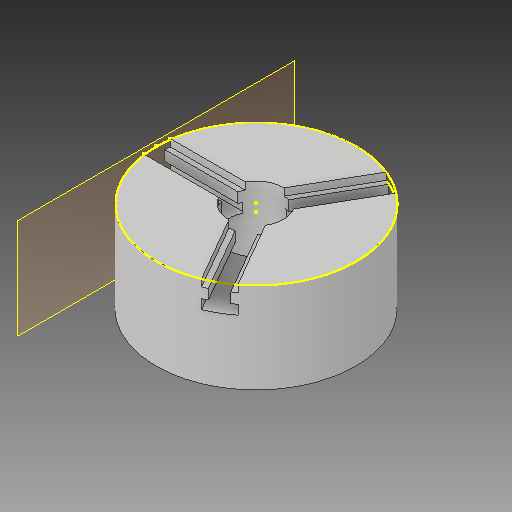
# Autodesk Inventor part: 3 jaww
Saved by Autodesk Inventor 2018 (Build 220112000, 112)
## iProperties
Created: 2017-06-20
Part Number: 3 jaww
Material: Generic
Document SubType Name: Modeling
Designer: M228854
Density: 1 g/cm^3
Appearance: Default
Author: M228854
Autodesk Inventor part; units mm, degrees
ref_plane "XZ Plane" through (0, 0, 0) normal (0, 1, 0) x (-1, 0, 0)
ref_plane "XY Plane" through (0, 0, 0) normal (0, 0, 1) x (1, 0, 0)
sketch "Sketch1" plane through (0, 0, 0) normal (0, 1, 0) x (-1, 0, 0)
  circle A0 centre (0, 0) radius 99.7
  constraints: 1 centre point, 1 coincident
extrude "Extrusion1" add sketch "Sketch1" along normal blind 90.9
sketch "Sketch2" plane through (0, 90.9, 0) normal (0, 1, 0) x (1, 0, 0)
  circle A0 centre (0, 0) radius 27.56
  dimension "d3" = 55.12
  constraints: 1 centre point, 1 coincident
  measures "d3" diameter of A0
extrude "Extrusion2" cut sketch "Sketch2" against normal blind 90.9
sketch "Sketch3" plane through (0, 90.9, 0) normal (0, 1, 0) x (1, 0, 0)
  circle A0 centre (0, 0) radius 99.7 projected
  line L0 (-99.7, 0) -> (-98.8062, 13.32)
  line L1 (-98.8062, 13.32) -> (-24.1274, 13.32)
  circle A1 centre (0, 0) radius 27.56 projected
  line L2 (-99.7, 0) -> (-98.8062, -13.32)
  line L3 (-98.8062, -13.32) -> (-24.1274, -13.32)
  line L4 (37.8676, -92.2287) -> (0.5282, -27.5549)
  line L5 (49.85, -86.3427) -> (37.8676, -92.2287)
  line L6 (49.85, -86.3427) -> (60.9386, -78.9087)
  line L7 (60.9386, -78.9087) -> (23.5992, -14.2349)
  line L8 (60.9386, 78.9087) -> (23.5992, 14.2349)
  line L9 (49.85, 86.3427) -> (60.9386, 78.9087)
  line L10 (49.85, 86.3427) -> (37.8676, 92.2287)
  line L11 (37.8676, 92.2287) -> (0.5282, 27.5549)
  line L12 (-24.1274, 13.32) -> (-24.1274, -13.32)
  line L13 (0.5282, 27.5549) -> (23.5992, 14.2349)
  line L14 (23.5992, -14.2349) -> (0.5282, -27.5549)
  dimension "d6" = 13.35
  dimension "d15" = 360
  constraints: 30 end point, 5 point on circle, 2 horizontal, 1 perpendicular, 1 vertical, 28 other
  measures "d6" distance of L0.start L0.end
extrude "Extrusion6" cut sketch "Sketch3" against normal blind 7.18 contours L8 A1 L11 L10 L9 | L6 L5 L4 A1 L7 | L13 A1 | A1 L14 | L1 A1 L3 L2 L0
sketch "Sketch7" plane through (49.85, 83.72, -86.3427) normal (-0.5568593, 0, 0.8306069) x (0.8306069, 0, 0.5568593)
  line L0 (13.35, 7.18) -> (0, 7.18) projected
  line L1 (13.35, 0) -> (13.35, 7.18) projected
  line L2 (0, 7.18) -> (13.35, 7.18)
  line L3 (13.35, 0) -> (18.3498, 0) projected
  line L4 (13.35, 7.18) -> (13.35, 0)
  line L5 (0, 7.18) -> (0, 0) projected
  line L6 (13.35, 0) -> (0, 0)
  line L7 (0, 0) -> (0, 6.2119)
  line L8 (0, 7.18) -> (-13.2303, 7.18) projected
  line L9 (-13.2303, 4.6736) -> (0, 7.18)
  line L10 (0, 7.18) -> (0, 0)
  line L11 (-13.2303, -2.9965) -> (-13.2303, 4.6736)
  line L12 (-13.2303, 0) -> (-13.2303, 7.18) projected
  point P0 (6.675, -83.72)
  constraints: 14 end point, 3 perpendicular, 2 collinear, 1 point on line
extrude "Extrusion7" cut sketch "Sketch7" against normal blind 10 contours L1 L6 L5 L0
sketch "Sketch8" plane through (37.8676, 83.72, -92.2287) normal (-0.440897, 0, 0.8975577) x (0.8975577, 0, 0.440897)
  line L0 (0, 0) -> (0, 7.18) projected
  line L1 (-4.9998, 0) -> (0, 0) projected
  line L2 (0, 7.18) -> (0, 0)
  line L3 (0, 0) -> (13.35, 0) projected
  line L4 (0, 0) -> (13.35, 0)
  line L5 (13.35, 7.18) -> (13.35, 0) projected
  line L6 (13.35, 0) -> (13.35, 7.18)
  line L7 (0, 7.18) -> (13.35, 7.18) projected
  line L8 (13.35, 7.18) -> (0, 7.18)
  line L9 (0, 7.18) -> (0, 4.7035)
  point P0 (6.675, -83.72)
  constraints: 10 end point, 3 collinear, 1 point on line, 1 vertical
extrude "Extrusion8" cut sketch "Sketch8" against normal blind 10
sketch "Sketch10" plane through (49.85, 83.72, 86.3427) normal (-0.440897, 0, -0.8975577) x (-0.8975577, 0, 0.440897)
  line L0 (0, 7.18) -> (13.35, 7.18) projected
  line L1 (13.35, 7.18) -> (18.3498, 7.18) projected
  line L2 (0, 7.18) -> (13.35, 7.18)
  line L3 (13.35, 0) -> (18.3498, 0) projected
  line L4 (13.35, 7.18) -> (13.35, 0)
  line L5 (0, 0) -> (13.35, 0) projected
  line L6 (13.35, 0) -> (0, 0)
  line L7 (0, 0) -> (0, 7.18)
  line L8 (0, 7.18) -> (0, 0) projected
  point P0 (6.675, -83.72)
  constraints: 8 end point, 2 collinear, 1 horizontal, 1 perpendicular
extrude "Extrusion9" cut sketch "Sketch10" against normal blind 10
sketch "Sketch11" plane through (60.9386, 83.72, 78.9087) normal (-0.5568593, 0, -0.8306069) x (-0.8306069, 0, 0.5568593)
  line L0 (-4.9998, 7.18) -> (0, 7.18) projected
  line L1 (96.1615, 7.18) -> (0, 7.18) projected
  line L2 (0, 7.18) -> (13.35, 7.18)
  line L3 (0, 0) -> (13.35, 0) projected
  line L4 (13.35, 7.18) -> (13.35, 0)
  line L5 (13.35, 0) -> (0, 0)
  line L6 (0, 0) -> (0, 7.18) projected
  line L7 (0, 0) -> (0, 7.18)
  point P0 (6.675, -83.72)
  constraints: 8 end point, 3 collinear, 1 perpendicular
extrude "Extrusion10" cut sketch "Sketch11" against normal blind 10
sketch "Sketch12" plane through (0, 90.9, 0) normal (0, 1, 0) x (1, 0, 0)
  arc A0 (37.8676, -92.2287) -> (60.9386, -78.9087) centre (0, 0) ccw projected
  arc A1 (-99.7, 0) -> (-98.8062, -13.32) centre (0, 0) ccw projected
  arc A2 (60.9386, 78.9087) -> (37.8676, 92.2287) centre (0, 0) ccw projected
  circle A3 centre (0, 0) radius 99.7 projected
  arc A4 (-98.8062, -13.32) -> (37.8676, -92.2287) centre (0, 0) ccw projected
  arc A5 (-98.8062, 13.32) -> (-99.7, 0) centre (0, 0) ccw projected
  arc A6 (37.8676, 92.2287) -> (-98.8062, 13.32) centre (0, 0) ccw projected
  arc A7 (60.9386, -78.9087) -> (60.9386, 78.9087) centre (0, 0) ccw projected
  point P0 (-99.7, 0)
sketch "Sketch13" plane through (0, 83.72, 0) normal (0, 1, 0) x (1, 0, 0)
  arc A0 (60.9386, 78.9087) -> (37.8676, 92.2287) centre (0, 0) ccw projected
ref_plane "Work Plane10" through (-99.7, 0, 0) normal (1, 0, 0) x (0, 1, 0)
sketch "Sketch16" plane through (-99.7, 0, 0) normal (1, 0, 0) x (0, 1, 0)
  line L0 (83.72, 0) -> (83.72, -13.32) projected
  line L1 (83.72, -8.22) -> (73.62, -8.22)
  line L2 (83.72, 13.32) -> (83.72, 0) projected
  line L3 (83.72, 8.22) -> (73.62, 8.22)
  line L4 (73.62, -8.22) -> (73.62, -13.32)
  line L5 (73.62, -13.32) -> (64.1, -13.32)
  line L6 (64.1, -13.32) -> (64.1, 13.32)
  line L7 (64.1, 13.32) -> (73.62, 13.32)
  line L8 (73.62, 13.32) -> (73.62, 8.22)
  line L9 (83.72, -8.22) -> (83.72, 8.22)
  point P0 (0, 0)
  dimension "d36" = 9.52
  constraints: 16 end point, 3 perpendicular, 3 point on line, 1 collinear, 1 parallel, 1 vertical
  measures "d36" distance of L4.end L5.end
extrude "Extrusion11" cut sketch "Sketch16" along normal blind 74.5875
sketch "Sketch18" plane through (-98.8062, 83.72, -13.32) normal (0.9977563, 0, 0.0669509) x (0.0669509, 0, -0.9977563)
  line L0 (0, 0) -> (0, 7.18) projected
  line L1 (0, 7.18) -> (0, 0)
  arc A0 (0, 0) -> (-2.79, 0) centre (-1.395, 0) ccw
  line L2 (-13.35, 0) -> (-21.5289, 0) projected
  line L3 (-2.79, 0) -> (-13.35, 0)
  arc A1 (-13.35, 2.7204) -> (-13.35, 0) centre (-13.35, 1.3602) ccw
  line L4 (-13.35, 2.7204) -> (-13.35, 7.18)
  line L5 (-19.298, 7.18) -> (9.1079, 7.18) projected
  point P0 (-6.675, -83.72)
  constraints: 6 end point, 4 point on circle, 2 centre point, 2 perpendicular, 2 tangent, 1 collinear, 1 point on line
extrude "Extrusion12" cut sketch "Sketch18" along normal blind 74.5875
sketch "Sketch20" plane through (-99.7, 0, 0) normal (1, 0, 0) x (0, 1, 0)
  line L0 (90.9, 0) -> (90.9, -13.32) projected
  line L1 (83.72, -13.32) -> (90.9, -13.32) projected
  line L2 (90.9, -13.32) -> (83.72, -13.32)
  line L3 (83.72, 8.22) -> (83.72, 13.32) projected
  line L4 (83.72, -13.32) -> (83.72, 13.32)
  line L5 (83.72, 13.32) -> (90.9, 13.32)
  line L6 (90.9, 13.32) -> (90.9, -13.32)
  point P0 (0, 0)
  constraints: 8 end point, 3 collinear
extrude "Extrusion13" cut sketch "Sketch20" along normal blind 10
pattern_circular "Circular Pattern1" count 3 over 360 about axis through (0, 90.9, 0) along (0, -1, 0) of "Extrusion11"
sketch "Sketch21" plane through (0, 0, 0) normal (0, -1, 0) x (1, 0, 0)
  arc A0 (-98.8062, -13.32) -> (37.8676, -92.2287) centre (0, 0) ccw projected
  circle A1 centre (-39.56, 0) radius 10
  circle A2 centre (19.78, -34.26) radius 10
  circle A3 centre (19.78, 34.26) radius 10
  point P0 (-25.1125, 13.32)
  dimension "d50" = 360
  constraints: 3 centre point, 7 other
extrude "Extrusion14" cut sketch "Sketch21" against normal blind 50
body "Solid1"
